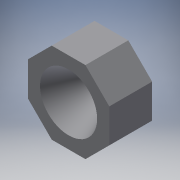
# Autodesk Inventor part: 03_Mikrolinse
Saved by Autodesk Inventor 2016 (Build 200138000, 138)
## iProperties
Created: 2016-07-31
Part Number: 03_Mikrolinse
Material: Generisch
Document SubType Name: Modeling
Designer: Bene
Density: 1 g/cm^3
Appearance: Vorgabe
Author: Bene
Autodesk Inventor part; units mm, degrees
ref_plane "YZ Plane" through (0, 0, 0) normal (1, 0, 0) x (0, 1, 0)
ref_plane "XZ Plane" through (0, 0, 0) normal (0, 1, 0) x (-1, 0, 0)
ref_plane "XY Plane" through (0, 0, 0) normal (0, 0, 1) x (1, 0, 0)
sketch "Skizze1" plane through (0, 0, 0) normal (0, 1, 0) x (-1, 0, 0)
  line L0 (4.75, 4.75) -> (-4.75, 4.75)
  line L1 (-4.75, 4.75) -> (-4.75, -4.75)
  line L2 (-4.75, -4.75) -> (4.75, -4.75)
  line L3 (4.75, -4.75) -> (4.75, 4.75)
  line L4 (4.75, 4.75) -> (-4.75, -4.75) construction
  line L5 (-4.75, 4.75) -> (4.75, -4.75) construction
  line L6 (0, 6.7175) -> (6.7175, 0)
  line L7 (6.7175, 0) -> (0, -6.7175)
  line L8 (0, -6.7175) -> (-6.7175, 0)
  line L9 (-6.7175, 0) -> (0, 6.7175)
  line L10 (0, 6.7175) -> (0, -6.7175) construction
  line L11 (6.7175, 0) -> (-6.7175, 0) construction
  point P0 (0, 0)
  point P1 (4.75, 1.9675)
  point P2 (4.75, -1.9675)
  point P3 (1.9675, -4.75)
  point P4 (-1.9675, -4.75)
  point P5 (-4.75, -1.9675)
  point P6 (-4.75, 1.9675)
  point P7 (-1.9675, 4.75)
  point P8 (1.9675, 4.75)
  dimension "d0" = 9.5
  dimension "d1" = 9.5
  dimension "d2" = 9.5
  dimension "d3" = 9.5
  constraints: 24 end point, 16 point on line, 4 midpoint, 4 parallel, 2 perpendicular, 1 horizontal
  measures "d0" distance of L2.end L1.end
  measures "d1" distance of L1.end L0.end
  measures "d2" distance of L6.start L6.end
  measures "d3" distance of L6.end L7.end
extrude "Extrusion1" add sketch "Skizze1" along normal blind 5 contours L6 L3 L7 L2 L8 L1 L9 L0
sketch "Skizze2" plane through (0, 5, 0) normal (0, 1, 0) x (1, 0, 0)
  circle A0 centre (0, 0) radius 1
  dimension "d6" = 2
  constraints: 1 centre point, 1 coincident
  measures "d6" diameter of A0
extrude "Extrusion2" cut sketch "Skizze2" against normal blind 5 draft 25
